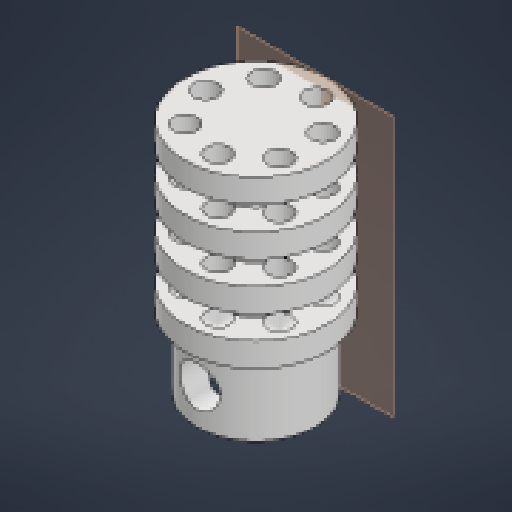
# Autodesk Inventor part: felga
Saved by Autodesk Inventor 2023 (Build 270158000, 158)
## iProperties
Created: 2024-02-27
Part Number: felga
Material: Generic
Document SubType Name: Modeling
Designer: Michał
Density: 1 g/cm^3
Appearance: Default
Author: Michał
Autodesk Inventor part; units mm, degrees
ref_plane "YZ Plane" through (0, 0, 0) normal (1, 0, 0) x (0, 1, 0)
ref_plane "XZ Plane" through (0, 0, 0) normal (0, 1, 0) x (-1, 0, 0)
sketch "Sketch5" plane through (0, 0, 0) normal (0, 0, 1) x (1, 0, 0)
  line L0 (0, 0) -> (0, 20)
  line L1 (0, 20) -> (6, 20)
  line L2 (6, 20) -> (6, 18)
  line L3 (6, 18) -> (3.5, 18)
  line L4 (3.5, 18) -> (3.5, 16)
  line L5 (3.5, 16) -> (6, 16)
  line L6 (6, 16) -> (6, 14)
  line L7 (6, 14) -> (3.5, 14)
  line L8 (3.5, 14) -> (3.5, 12)
  line L9 (3.5, 12) -> (6, 12)
  line L10 (6, 12) -> (6, 10)
  line L11 (6, 10) -> (3.5, 10)
  line L12 (3.5, 10) -> (3.5, 8)
  line L13 (3.5, 8) -> (6, 8)
  line L14 (6, 8) -> (6, 6)
  line L15 (6, 6) -> (5, 6)
  line L16 (5, 6) -> (5, 0)
  line L17 (5, 0) -> (0, 0)
  line L18 (0, 12) -> (3, 12)
  line L19 (3, 12) -> (3, 0)
  dimension "d32" = 2
  dimension "d33" = 2
  dimension "d36" = 4
  dimension "d41" = 2.5
  dimension "d42" = 6
  dimension "d43" = 20
  dimension "d44" = 5
  dimension "d46" = 3
  dimension "d47" = 12
  constraints: 40 end point, 7 perpendicular, 4 vertical, 2 collinear, 2 horizontal, 2 point on line, 18 other
  measures "d32" distance of L3.end L4.end
  measures "d33" distance of L1.end L2.end
  measures "d36" distance of L1.end L6.start
  measures "d41" distance of L2.end L3.end
  measures "d42" distance of L0.end L1.end
  measures "d43" distance between parallel lines of L1 L17
  measures "d44" distance between parallel lines of L0 L16
  measures "d46" distance between parallel lines of L19 L0
  measures "d47" distance between parallel lines of L17 L18
revolve "Revolution2" add sketch "Sketch5" angle 360 about axis through (0, 0, 0) along (0, 1, 0) contours L0 L1 L2 L3 L4 L5 L6 L7 L8 L9 L10 L11 L12 L13 L14 L15 L16 L17 L19 L18
sketch "Sketch6" plane through (0, 20, 0) normal (0, 1, 0) x (1, 0, 0)
  circle A0 centre (0, 0) radius 4.25 construction
  point P0 (-4.25, 0)
  point P1 (-2.6498, -3.3228)
  point P2 (0.9457, -4.1434)
  point P3 (3.8291, -1.844)
  point P4 (3.8291, 1.844)
  point P5 (0.9457, 4.1434)
  point P6 (-2.6498, 3.3228)
  dimension "d48" = 8.5
  dimension "d51" = 360
  constraints: 2 horizontal alignment, 1 coincident, 10 other
hole "Hole3" at (-4.25, 20, 0) at (-2.6498, 20, 3.3228) at (0.9457, 20, 4.1434) at (3.8291, 20, 1.844) at (3.8291, 20, -1.844) at (0.9457, 20, -4.1434) at (-2.6498, 20, -3.3228) direction (0, -1, 0) diameter 2 depth 12 tip angle 118
ref_plane "Work Plane4" through (0, 3, -5) normal (0, 0, 1) x (1, 0, 0)
sketch "Sketch7" plane through (0, 3, -5) normal (0, 0, 1) x (1, 0, 0)
  line L0 (0, -3) -> (0, 3) construction
  line L1 (6, 3) -> (-6, 3) construction
  point P0 (0, 0)
  constraints: 2 end point, 2 midpoint
hole "Hole4" at (0, 3, -5) direction (0, 0, 1) diameter 3.4 end through all counterbore diameter 5.7 counterbore depth 1.5 clearance for "Slotted Cheese Head Screw ISO 1207" size "M3" standard "ISO"
equation "\"d36\" = d32 + d33"
body "Solid2"
